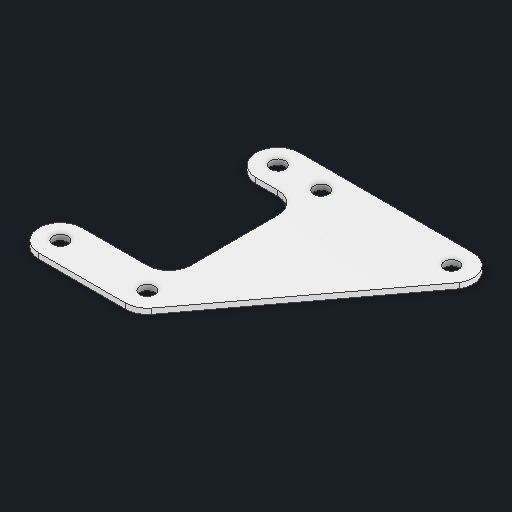
# Autodesk Inventor part: gusset
Saved by Autodesk Inventor 2024 (Build 280153000, 153)
## iProperties
Created: 2024-03-02
Part Number: gusset
Material: Acetal Resin, White
Document SubType Name: Modeling
Designer: Averey Ku
Density: 1.425 g/cm^3
Appearance: Smooth - White
d0: 0.250 in
d4: 0.165 in
Author: Averey Ku
Autodesk Inventor part; units mm, degrees
ref_plane "YZ Plane" through (0, 0, 0) normal (1, 0, 0) x (0, 1, 0)
ref_plane "XZ Plane" through (0, 0, 0) normal (0, 1, 0) x (-1, 0, 0)
ref_plane "XY Plane" through (0, 0, 0) normal (0, 0, 1) x (1, 0, 0)
sketch "main" plane through (0, 0, 0) normal (0, 0, 1) x (1, 0, 0)
  circle A0 centre (33.5416, 32.0006) radius 2.1844
  line L0 (8.1416, 38.3506) -> (33.5416, 38.3506)
  line L1 (33.5416, 25.6506) -> (14.4916, 25.6506)
  arc A1 (33.5416, 25.6506) -> (33.5416, 38.3506) centre (33.5416, 32.0006) ccw
  circle A2 centre (8.1416, 32.0006) radius 2.1844
  arc A3 (14.4916, 25.6506) -> (8.1416, 19.3006) centre (14.4916, 19.3006) ccw
  arc A4 (8.1416, 38.3506) -> (2.462, 34.8404) centre (8.1416, 32.0006) ccw
  line L2 (8.1416, -6.0994) -> (8.1416, 19.3006)
  arc A5 (8.1416, -6.0994) -> (14.4916, -12.4494) centre (14.4916, -6.0994) ccw
  circle A6 centre (8.1416, -18.7994) radius 2.1844
  line L3 (14.4916, -12.4494) -> (20.8416, -12.4494)
  line L4 (-29.9584, -25.1494) -> (20.8416, -25.1494)
  arc A7 (20.8416, -25.1494) -> (20.8416, -12.4494) centre (20.8416, -18.7994) ccw
  circle A8 centre (20.8416, -18.7994) radius 2.1844
  circle A9 centre (-29.9584, -18.7994) radius 2.0955
  arc A10 (-34.5524, -14.4156) -> (-29.9584, -25.1494) centre (-29.9584, -18.7994) ccw
  line L5 (-35.4577, -15.6244) -> (3.0589, 35.807)
  point P0 (9.5067, 8.1196)
  point P1 (8.1416, 25.6506)
  point P2 (8.1416, -12.4494)
  dimension "d0" = 6.35
  dimension "d4" = 4.191
  measures "d0" radius of A3
  measures "d4" diameter of A9
sketch "Sketch1" plane through (0, 0, 0) normal (0, 1, 0) x (-1, 0, 0)
  circle A0 centre (0, 0) radius 2.1844
  line L0 (-25.4, 6.35) -> (0, 6.35)
  line L1 (0, -6.35) -> (-19.05, -6.35)
  arc A1 (0, -6.35) -> (0, 6.35) centre (0, 0) ccw
  circle A2 centre (-25.4, 0) radius 2.1844
  arc A3 (-19.05, -6.35) -> (-25.4, -12.7) centre (-19.05, -12.7) ccw
  arc A4 (-25.4, 6.35) -> (-31.0796, 2.8398) centre (-25.4, 0) ccw
  line L2 (-25.4, -38.1) -> (-25.4, -12.7)
  arc A5 (-25.4, -38.1) -> (-19.05, -44.45) centre (-19.05, -38.1) ccw
  circle A6 centre (-25.4, -50.8) radius 2.1844
  line L3 (-19.05, -44.45) -> (-12.7, -44.45)
  line L4 (-63.5, -57.15) -> (-12.7, -57.15)
  arc A7 (-12.7, -57.15) -> (-12.7, -44.45) centre (-12.7, -50.8) ccw
  circle A8 centre (-12.7, -50.8) radius 2.1844
  circle A9 centre (-63.5, -50.8) radius 2.0955
  arc A10 (-68.094, -46.4162) -> (-63.5, -57.15) centre (-63.5, -50.8) ccw
  line L5 (-68.9993, -47.625) -> (-30.4827, 3.8064)
  constraints: 1 other
extrude "Extrusion1" add sketch "Sketch1" along normal blind 1.5875 contours L0 A1 L1 A3 L2 A5 L3 A7 L4 A10 L5 A4
body "Solid1"
